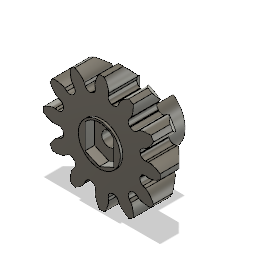
PinionGear (Autodesk Fusion 360 design; units mm, degrees)
description: Spur Gear; Module: 1.75; Num Teeth: 12; Pressure Angle: 20.0; Backlash: 0.00 mm
Autodesk Fusion 360 part; units mm, degrees
(part 1 of 3)
sketch "Sketch1" plane through (0, 0, 0) normal (0, 0, 1) x (1, 0, 0) in component "Spur Gear (12 teeth)"
  circle A0 centre (0, 0) radius 8.3492
  circle A1 centre (0, 0) radius 3
extrude "Extrude1" add sketch "Sketch1" along normal blind 6 in component "Spur Gear (12 teeth)"
sketch "Sketch2" plane through (0, 0, 0) normal (0, 0, 1) x (1, 0, 0) in component "Spur Gear (12 teeth)"
  spline S0 degree 5 poles (9.7621, -1.4335) (9.7691, -1.4345) (9.783, -1.4364) (9.8041, -1.4384) (9.8322, -1.4399) (9.8676, -1.44) (9.903, -1.4389) (9.9385, -1.437) (9.9741, -1.4347) (10.0097, -1.4321) (10.0453, -1.4292) (10.081, -1.4258) (10.1167, -1.422) (10.1525, -1.4175) (10.1882, -1.4124) (10.224, -1.4067) (10.2599, -1.4005) (10.2957, -1.3939) (10.3316, -1.387) (10.3674, -1.3797) (10.4033, -1.3721) (10.4391, -1.364) (10.475, -1.3556) (10.5109, -1.3469) (10.5468, -1.3377) (10.5826, -1.3281) (10.6185, -1.3182) (10.6543, -1.3079) (10.6902, -1.2973) (10.726, -1.2864) (10.7619, -1.2752) (10.7977, -1.2636) (10.8335, -1.2517) (10.8693, -1.2395) (10.905, -1.227) (10.9408, -1.2141) (10.9765, -1.2009) (11.0122, -1.1875) (11.0479, -1.1737) (11.0835, -1.1597) (11.1191, -1.1453) (11.1547, -1.1307) (11.1903, -1.1158) (11.2259, -1.1005) (11.2614, -1.085) (11.2968, -1.0692) (11.3323, -1.0532) (11.3677, -1.0368) (11.4031, -1.0202) (11.4384, -1.0033) (11.4737, -0.9861) (11.5089, -0.9687) (11.5441, -0.951) (11.5793, -0.933) (11.6144, -0.9148) (11.6495, -0.8963) (11.6845, -0.8775) (11.7195, -0.8585) (11.7545, -0.8392) (11.7894, -0.8197) (11.8242, -0.7999) (11.859, -0.7799) (11.8937, -0.7596) (11.9284, -0.7391) (11.963, -0.7183) (11.9976, -0.6972) (12.0321, -0.6759) (12.0666, -0.6544) (12.101, -0.6327) (12.1353, -0.6106) (12.1696, -0.5884) (12.197, -0.5704) (12.2175, -0.5568) (12.2311, -0.5477) (12.238, -0.5431) knots 0 0 0 0 0 0 0.01428571 0.02857143 0.04285714 0.05714286 0.07142857 0.08571429 0.1 0.11428571 0.12857143 0.14285714 0.15714286 0.17142857 0.18571429 0.2 0.21428571 0.22857143 0.24285714 0.25714286 0.27142857 0.28571429 0.3 0.31428571 0.32857143 0.34285714 0.35714286 0.37142857 0.38571429 0.4 0.41428571 0.42857143 0.44285714 0.45714286 0.47142857 0.48571429 0.5 0.51428571 0.52857143 0.54285714 0.55714286 0.57142857 0.58571429 0.6 0.61428571 0.62857143 0.64285714 0.65714286 0.67142857 0.68571429 0.7 0.71428571 0.72857143 0.74285714 0.75714286 0.77142857 0.78571429 0.8 0.81428571 0.82857143 0.84285714 0.85714286 0.87142857 0.88571429 0.9 0.91428571 0.92857143 0.94285714 0.95714286 0.97142857 0.98571429 1 1 1 1 1 1
  spline S1 degree 5 poles (9.7621, 1.4335) (9.7691, 1.4345) (9.783, 1.4364) (9.8041, 1.4384) (9.8322, 1.4399) (9.8676, 1.44) (9.903, 1.4389) (9.9385, 1.437) (9.9741, 1.4347) (10.0097, 1.4321) (10.0453, 1.4292) (10.081, 1.4258) (10.1167, 1.422) (10.1525, 1.4175) (10.1882, 1.4124) (10.224, 1.4067) (10.2599, 1.4005) (10.2957, 1.3939) (10.3316, 1.387) (10.3674, 1.3797) (10.4033, 1.3721) (10.4391, 1.364) (10.475, 1.3556) (10.5109, 1.3469) (10.5468, 1.3377) (10.5826, 1.3281) (10.6185, 1.3182) (10.6543, 1.3079) (10.6902, 1.2973) (10.726, 1.2864) (10.7619, 1.2752) (10.7977, 1.2636) (10.8335, 1.2517) (10.8693, 1.2395) (10.905, 1.227) (10.9408, 1.2141) (10.9765, 1.2009) (11.0122, 1.1875) (11.0479, 1.1737) (11.0835, 1.1597) (11.1191, 1.1453) (11.1547, 1.1307) (11.1903, 1.1158) (11.2259, 1.1005) (11.2614, 1.085) (11.2968, 1.0692) (11.3323, 1.0532) (11.3677, 1.0368) (11.4031, 1.0202) (11.4384, 1.0033) (11.4737, 0.9861) (11.5089, 0.9687) (11.5441, 0.951) (11.5793, 0.933) (11.6144, 0.9148) (11.6495, 0.8963) (11.6845, 0.8775) (11.7195, 0.8585) (11.7545, 0.8392) (11.7894, 0.8197) (11.8242, 0.7999) (11.859, 0.7799) (11.8937, 0.7596) (11.9284, 0.7391) (11.963, 0.7183) (11.9976, 0.6972) (12.0321, 0.6759) (12.0666, 0.6544) (12.101, 0.6327) (12.1353, 0.6106) (12.1696, 0.5884) (12.197, 0.5704) (12.2175, 0.5568) (12.2311, 0.5477) (12.238, 0.5431) knots 0 0 0 0 0 0 0.01428571 0.02857143 0.04285714 0.05714286 0.07142857 0.08571429 0.1 0.11428571 0.12857143 0.14285714 0.15714286 0.17142857 0.18571429 0.2 0.21428571 0.22857143 0.24285714 0.25714286 0.27142857 0.28571429 0.3 0.31428571 0.32857143 0.34285714 0.35714286 0.37142857 0.38571429 0.4 0.41428571 0.42857143 0.44285714 0.45714286 0.47142857 0.48571429 0.5 0.51428571 0.52857143 0.54285714 0.55714286 0.57142857 0.58571429 0.6 0.61428571 0.62857143 0.64285714 0.65714286 0.67142857 0.68571429 0.7 0.71428571 0.72857143 0.74285714 0.75714286 0.77142857 0.78571429 0.8 0.81428571 0.82857143 0.84285714 0.85714286 0.87142857 0.88571429 0.9 0.91428571 0.92857143 0.94285714 0.95714286 0.97142857 0.98571429 1 1 1 1 1 1
  arc A0 (12.238, -0.5431) -> (12.238, 0.5431) centre (0, 0) ccw
  line L0 (8.2507, -1.213) -> (9.7621, -1.4335)
  line L1 (8.2507, 1.213) -> (9.7621, 1.4335)
  line L2 (8.2507, -1.213) -> (8.2507, 1.213)
  point P0 (9.9336, -1.4372)
  point P1 (10.1076, -1.4229)
  point P2 (10.2831, -1.3962)
  point P3 (10.4598, -1.3592)
  point P4 (10.6372, -1.3128)
  point P5 (10.8153, -1.2577)
  point P6 (10.9937, -1.1944)
  point P7 (11.1723, -1.1233)
  point P8 (11.3509, -1.0445)
  point P9 (11.5293, -0.9584)
  point P10 (11.7074, -0.8651)
  point P11 (11.885, -0.7647)
  point P12 (12.0619, -0.6573)
  point P13 (9.9336, 1.4372)
  point P14 (10.1076, 1.4229)
  point P15 (10.2831, 1.3962)
  point P16 (10.4598, 1.3592)
  point P17 (10.6372, 1.3128)
  point P18 (10.8153, 1.2577)
  point P19 (10.9937, 1.1944)
  point P20 (11.1723, 1.1233)
  point P21 (11.3509, 1.0445)
  point P22 (11.5293, 0.9584)
  point P23 (11.7074, 0.8651)
  point P24 (11.885, 0.7647)
  point P25 (12.0619, 0.6573)
extrude "Extrude2" add sketch "Sketch2" along normal blind 6 in component "Spur Gear (12 teeth)"
fillet "Fillet1" radius 1 2 edges at (8.2604, -1.2145, 3) (8.2604, 1.2145, 3) in component "Spur Gear (12 teeth)"
pattern_circular "C-Pattern1" count 12 over 360 about axis through (0, 0, 0) along (0, 0, 1) of "Extrude2", "Fillet1" in component "Spur Gear (12 teeth)"
sketch "Sketch3" plane through (0, 0, 0) normal (0, 0, 1) x (1, 0, 0) in component "Spur Gear (12 teeth)"
  circle A0 centre (0, 0) radius 10.5 construction
  circle A1 centre (0, 0) radius 12.25 construction
  point P0 (0.5431, 12.238)
  constraint concentric A0 A1
  constraint coincident A1 P0
sketch "Sketch1 (2)" plane through (0, 0, 0) normal (0, 1, 0) x (1, 0, 0)
  line L0 (-12.25, 0) -> (12.25, 0) construction
  line L1 (12.25, 0) -> (12.25, -2)
  line L2 (12.25, -2) -> (10.25, 0)
  line L3 (0, 0) -> (0, 10) construction
  line L4 (10.25, 0) -> (12.25, 0)
  dimension "d8" = 2
  constraint coincident L0.end L1.start
  constraint perpendicular L0 L1
  constraint coincident L0 L2.end
  constraint coincident L3.start origin
  constraint perpendicular L0 L3
  constraint equal L1 L4
  measures "d8" distance of L0.end L1.end
revolve "Revolve1" cut sketch "Sketch1 (2)" angle 360 about axis through (0, 0, 0) along (0, 0, -1) in component "Spur Gear (12 teeth)"
sketch "Sketch3 (2)" plane through (0, 0, 0) normal (0, 0, -1) x (-1, 0, 0)
  arc A0 (-9.5002, -3.8482) -> (-8.0827, -6.3033) centre (0, 0) ccw
  spline S0 degree 5 poles (-7.7374, -6.1225) (-7.743, -6.1269) (-7.7542, -6.1354) (-7.7714, -6.1477) (-7.795, -6.1631) (-7.8255, -6.1809) (-7.8568, -6.1976) (-7.8885, -6.2138) (-7.9205, -6.2295) (-7.9526, -6.2451) (-7.9849, -6.2604) (-8.0173, -6.2752) (-8.0434, -6.2868) (-8.0631, -6.2952) (-8.0763, -6.3006) (-8.0827, -6.3033) knots 0 0 0 0 0 0 0.014286 0.028571 0.042857 0.057143 0.071429 0.085714 0.1 0.114286 0.128571 0.142857 0.156761 0.156761 0.156761 0.156761 0.156761 0.156761
  line L0 (-7.7374, -6.1225) -> (-7.2884, -5.7679)
  arc A1 (-5.9553, -5.8518) -> (-7.2884, -5.7679) centre (-6.6686, -6.5526) ccw
  arc A2 (-5.9553, -5.8518) -> (-5.8518, -5.9553) centre (0, 0) ccw
  arc A3 (-5.7679, -7.2884) -> (-5.8518, -5.9553) centre (-6.5526, -6.6686) ccw
  line L1 (-5.7679, -7.2884) -> (-6.1225, -7.7374)
  spline S1 degree 5 poles (-6.1225, -7.7374) (-6.1269, -7.743) (-6.1354, -7.7542) (-6.1477, -7.7714) (-6.1631, -7.795) (-6.1809, -7.8255) (-6.1976, -7.8568) (-6.2138, -7.8885) (-6.2295, -7.9205) (-6.2451, -7.9526) (-6.2604, -7.9849) (-6.2752, -8.0173) (-6.2868, -8.0434) (-6.2952, -8.0631) (-6.3006, -8.0763) (-6.3033, -8.0827) knots 0 0 0 0 0 0 0.014286 0.028571 0.042857 0.057143 0.071429 0.085714 0.1 0.114286 0.128571 0.142857 0.156761 0.156761 0.156761 0.156761 0.156761 0.156761
  arc A4 (-6.3033, -8.0827) -> (-3.8482, -9.5002) centre (0, 0) ccw
  spline S2 degree 5 poles (-3.6396, -9.171) (-3.6422, -9.1775) (-3.6476, -9.1905) (-3.6563, -9.2098) (-3.6691, -9.2349) (-3.6867, -9.2656) (-3.7054, -9.2957) (-3.7248, -9.3255) (-3.7446, -9.3552) (-3.7646, -9.3847) (-3.785, -9.4141) (-3.8056, -9.4432) (-3.8224, -9.4662) (-3.8353, -9.4833) (-3.8439, -9.4946) (-3.8482, -9.5002) knots 0 0 0 0 0 0 0.014286 0.028571 0.042857 0.057143 0.071429 0.085714 0.1 0.114286 0.128571 0.142857 0.156761 0.156761 0.156761 0.156761 0.156761 0.156761
  line L2 (-3.6396, -9.171) -> (-3.428, -8.6393)
  arc A5 (-2.2316, -8.0454) -> (-3.428, -8.6393) centre (-2.4989, -9.0091) ccw
  arc A6 (-2.2316, -8.0454) -> (-2.0901, -8.0834) centre (0, 0) ccw
  arc A7 (-1.3509, -9.1959) -> (-2.0901, -8.0834) centre (-2.3404, -9.0515) ccw
  line L3 (-1.3509, -9.1959) -> (-1.4335, -9.7621)
  spline S3 degree 5 poles (-1.4335, -9.7621) (-1.4345, -9.7691) (-1.4364, -9.783) (-1.4384, -9.8041) (-1.4399, -9.8322) (-1.44, -9.8676) (-1.4389, -9.903) (-1.437, -9.9385) (-1.4347, -9.9741) (-1.4321, -10.0097) (-1.4292, -10.0453) (-1.4258, -10.0808) (-1.4228, -10.1092) (-1.4202, -10.1304) (-1.4184, -10.1446) (-1.4175, -10.1515) knots 0 0 0 0 0 0 0.014286 0.028571 0.042857 0.057143 0.071429 0.085714 0.1 0.114286 0.128571 0.142857 0.156761 0.156761 0.156761 0.156761 0.156761 0.156761
  arc A8 (-1.4175, -10.1515) -> (1.4175, -10.1515) centre (0, 0) ccw
  spline S4 degree 5 poles (1.4335, -9.7621) (1.4345, -9.7691) (1.4364, -9.783) (1.4384, -9.8041) (1.4399, -9.8322) (1.44, -9.8676) (1.4389, -9.903) (1.437, -9.9385) (1.4347, -9.9741) (1.4321, -10.0097) (1.4292, -10.0453) (1.4258, -10.0808) (1.4228, -10.1092) (1.4202, -10.1304) (1.4184, -10.1446) (1.4175, -10.1515) knots 0 0 0 0 0 0 0.014286 0.028571 0.042857 0.057143 0.071429 0.085714 0.1 0.114286 0.128571 0.142857 0.156761 0.156761 0.156761 0.156761 0.156761 0.156761
  line L4 (1.4335, -9.7621) -> (1.3509, -9.1959)
  arc A9 (2.0901, -8.0834) -> (1.3509, -9.1959) centre (2.3404, -9.0515) ccw
  arc A10 (2.0901, -8.0834) -> (2.2316, -8.0454) centre (0, 0) ccw
  arc A11 (3.428, -8.6393) -> (2.2316, -8.0454) centre (2.4989, -9.0091) ccw
  line L5 (3.428, -8.6393) -> (3.6396, -9.171)
  spline S5 degree 5 poles (3.6396, -9.171) (3.6422, -9.1775) (3.6476, -9.1905) (3.6563, -9.2098) (3.6691, -9.2349) (3.6867, -9.2656) (3.7054, -9.2957) (3.7248, -9.3255) (3.7446, -9.3552) (3.7646, -9.3847) (3.785, -9.4141) (3.8056, -9.4432) (3.8224, -9.4662) (3.8353, -9.4833) (3.8439, -9.4946) (3.8482, -9.5002) knots 0 0 0 0 0 0 0.014286 0.028571 0.042857 0.057143 0.071429 0.085714 0.1 0.114286 0.128571 0.142857 0.156761 0.156761 0.156761 0.156761 0.156761 0.156761
  arc A12 (3.8482, -9.5002) -> (6.3033, -8.0827) centre (0, 0) ccw
  spline S6 degree 5 poles (6.1225, -7.7374) (6.1269, -7.743) (6.1354, -7.7542) (6.1477, -7.7714) (6.1631, -7.795) (6.1809, -7.8255) (6.1976, -7.8568) (6.2138, -7.8885) (6.2295, -7.9205) (6.2451, -7.9526) (6.2604, -7.9849) (6.2752, -8.0173) (6.2868, -8.0434) (6.2952, -8.0631) (6.3006, -8.0763) (6.3033, -8.0827) knots 0 0 0 0 0 0 0.014286 0.028571 0.042857 0.057143 0.071429 0.085714 0.1 0.114286 0.128571 0.142857 0.156761 0.156761 0.156761 0.156761 0.156761 0.156761
  line L6 (6.1225, -7.7374) -> (5.7679, -7.2884)
  arc A13 (5.8518, -5.9553) -> (5.7679, -7.2884) centre (6.5526, -6.6686) ccw
  arc A14 (5.8518, -5.9553) -> (5.9553, -5.8518) centre (0, 0) ccw
  arc A15 (7.2884, -5.7679) -> (5.9553, -5.8518) centre (6.6686, -6.5526) ccw
  line L7 (7.2884, -5.7679) -> (7.7374, -6.1225)
  spline S7 degree 5 poles (7.7374, -6.1225) (7.743, -6.1269) (7.7542, -6.1354) (7.7714, -6.1477) (7.795, -6.1631) (7.8255, -6.1809) (7.8568, -6.1976) (7.8885, -6.2138) (7.9205, -6.2295) (7.9526, -6.2451) (7.9849, -6.2604) (8.0173, -6.2752) (8.0434, -6.2868) (8.0631, -6.2952) (8.0763, -6.3006) (8.0827, -6.3033) knots 0 0 0 0 0 0 0.014286 0.028571 0.042857 0.057143 0.071429 0.085714 0.1 0.114286 0.128571 0.142857 0.156761 0.156761 0.156761 0.156761 0.156761 0.156761
  arc A16 (8.0827, -6.3033) -> (9.5002, -3.8482) centre (0, 0) ccw
  spline S8 degree 5 poles (9.171, -3.6396) (9.1775, -3.6422) (9.1905, -3.6476) (9.2098, -3.6563) (9.2349, -3.6691) (9.2656, -3.6867) (9.2957, -3.7054) (9.3255, -3.7248) (9.3552, -3.7446) (9.3847, -3.7646) (9.4141, -3.785) (9.4432, -3.8056) (9.4662, -3.8224) (9.4833, -3.8353) (9.4946, -3.8439) (9.5002, -3.8482) knots 0 0 0 0 0 0 0.014286 0.028571 0.042857 0.057143 0.071429 0.085714 0.1 0.114286 0.128571 0.142857 0.156761 0.156761 0.156761 0.156761 0.156761 0.156761
  line L8 (9.171, -3.6396) -> (8.6393, -3.428)
  arc A17 (8.0454, -2.2316) -> (8.6393, -3.428) centre (9.0091, -2.4989) ccw
  arc A18 (8.0454, -2.2316) -> (8.0834, -2.0901) centre (0, 0) ccw
  arc A19 (9.1959, -1.3509) -> (8.0834, -2.0901) centre (9.0515, -2.3404) ccw
  line L9 (9.1959, -1.3509) -> (9.7621, -1.4335)
  spline S9 degree 5 poles (9.7621, -1.4335) (9.7691, -1.4345) (9.783, -1.4364) (9.8041, -1.4384) (9.8322, -1.4399) (9.8676, -1.44) (9.903, -1.4389) (9.9385, -1.437) (9.9741, -1.4347) (10.0097, -1.4321) (10.0453, -1.4292) (10.0808, -1.4258) (10.1092, -1.4228) (10.1304, -1.4202) (10.1446, -1.4184) (10.1515, -1.4175) knots 0 0 0 0 0 0 0.014286 0.028571 0.042857 0.057143 0.071429 0.085714 0.1 0.114286 0.128571 0.142857 0.156761 0.156761 0.156761 0.156761 0.156761 0.156761
  arc A20 (10.1515, -1.4175) -> (10.1515, 1.4175) centre (0, 0) ccw
  spline S10 degree 5 poles (9.7621, 1.4335) (9.7691, 1.4345) (9.783, 1.4364) (9.8041, 1.4384) (9.8322, 1.4399) (9.8676, 1.44) (9.903, 1.4389) (9.9385, 1.437) (9.9741, 1.4347) (10.0097, 1.4321) (10.0453, 1.4292) (10.0808, 1.4258) (10.1092, 1.4228) (10.1304, 1.4202) (10.1446, 1.4184) (10.1515, 1.4175) knots 0 0 0 0 0 0 0.014286 0.028571 0.042857 0.057143 0.071429 0.085714 0.1 0.114286 0.128571 0.142857 0.156761 0.156761 0.156761 0.156761 0.156761 0.156761
  line L10 (9.7621, 1.4335) -> (9.1959, 1.3509)
  arc A21 (8.0834, 2.0901) -> (9.1959, 1.3509) centre (9.0515, 2.3404) ccw
  arc A22 (8.0834, 2.0901) -> (8.0454, 2.2316) centre (0, 0) ccw
  arc A23 (8.6393, 3.428) -> (8.0454, 2.2316) centre (9.0091, 2.4989) ccw
  line L11 (8.6393, 3.428) -> (9.171, 3.6396)
  spline S11 degree 5 poles (9.171, 3.6396) (9.1775, 3.6422) (9.1905, 3.6476) (9.2098, 3.6563) (9.2349, 3.6691) (9.2656, 3.6867) (9.2957, 3.7054) (9.3255, 3.7248) (9.3552, 3.7446) (9.3847, 3.7646) (9.4141, 3.785) (9.4432, 3.8056) (9.4662, 3.8224) (9.4833, 3.8353) (9.4946, 3.8439) (9.5002, 3.8482) knots 0 0 0 0 0 0 0.014286 0.028571 0.042857 0.057143 0.071429 0.085714 0.1 0.114286 0.128571 0.142857 0.156761 0.156761 0.156761 0.156761 0.156761 0.156761
  arc A24 (9.5002, 3.8482) -> (8.0827, 6.3033) centre (0, 0) ccw
  spline S12 degree 5 poles (7.7374, 6.1225) (7.743, 6.1269) (7.7542, 6.1354) (7.7714, 6.1477) (7.795, 6.1631) (7.8255, 6.1809) (7.8568, 6.1976) (7.8885, 6.2138) (7.9205, 6.2295) (7.9526, 6.2451) (7.9849, 6.2604) (8.0173, 6.2752) (8.0434, 6.2868) (8.0631, 6.2952) (8.0763, 6.3006) (8.0827, 6.3033) knots 0 0 0 0 0 0 0.014286 0.028571 0.042857 0.057143 0.071429 0.085714 0.1 0.114286 0.128571 0.142857 0.156761 0.156761 0.156761 0.156761 0.156761 0.156761
  line L12 (7.7374, 6.1225) -> (7.2884, 5.7679)
  arc A25 (5.9553, 5.8518) -> (7.2884, 5.7679) centre (6.6686, 6.5526) ccw
  arc A26 (5.9553, 5.8518) -> (5.8518, 5.9553) centre (0, 0) ccw
  arc A27 (5.7679, 7.2884) -> (5.8518, 5.9553) centre (6.5526, 6.6686) ccw
  line L13 (5.7679, 7.2884) -> (6.1225, 7.7374)
  spline S13 degree 5 poles (6.1225, 7.7374) (6.1269, 7.743) (6.1354, 7.7542) (6.1477, 7.7714) (6.1631, 7.795) (6.1809, 7.8255) (6.1976, 7.8568) (6.2138, 7.8885) (6.2295, 7.9205) (6.2451, 7.9526) (6.2604, 7.9849) (6.2752, 8.0173) (6.2868, 8.0434) (6.2952, 8.0631) (6.3006, 8.0763) (6.3033, 8.0827) knots 0 0 0 0 0 0 0.014286 0.028571 0.042857 0.057143 0.071429 0.085714 0.1 0.114286 0.128571 0.142857 0.156761 0.156761 0.156761 0.156761 0.156761 0.156761
  arc A28 (6.3033, 8.0827) -> (3.8482, 9.5002) centre (0, 0) ccw
  spline S14 degree 5 poles (3.6396, 9.171) (3.6422, 9.1775) (3.6476, 9.1905) (3.6563, 9.2098) (3.6691, 9.2349) (3.6867, 9.2656) (3.7054, 9.2957) (3.7248, 9.3255) (3.7446, 9.3552) (3.7646, 9.3847) (3.785, 9.4141) (3.8056, 9.4432) (3.8224, 9.4662) (3.8353, 9.4833) (3.8439, 9.4946) (3.8482, 9.5002) knots 0 0 0 0 0 0 0.014286 0.028571 0.042857 0.057143 0.071429 0.085714 0.1 0.114286 0.128571 0.142857 0.156761 0.156761 0.156761 0.156761 0.156761 0.156761
  line L14 (3.6396, 9.171) -> (3.428, 8.6393)
  arc A29 (2.2316, 8.0454) -> (3.428, 8.6393) centre (2.4989, 9.0091) ccw
  arc A30 (2.2316, 8.0454) -> (2.0901, 8.0834) centre (0, 0) ccw
  arc A31 (1.3509, 9.1959) -> (2.0901, 8.0834) centre (2.3404, 9.0515) ccw
  line L15 (1.3509, 9.1959) -> (1.4335, 9.7621)
  spline S15 degree 5 poles (1.4335, 9.7621) (1.4345, 9.7691) (1.4364, 9.783) (1.4384, 9.8041) (1.4399, 9.8322) (1.44, 9.8676) (1.4389, 9.903) (1.437, 9.9385) (1.4347, 9.9741) (1.4321, 10.0097) (1.4292, 10.0453) (1.4258, 10.0808) (1.4228, 10.1092) (1.4202, 10.1304) (1.4184, 10.1446) (1.4175, 10.1515) knots 0 0 0 0 0 0 0.014286 0.028571 0.042857 0.057143 0.071429 0.085714 0.1 0.114286 0.128571 0.142857 0.156761 0.156761 0.156761 0.156761 0.156761 0.156761
  arc A32 (1.4175, 10.1515) -> (-1.4175, 10.1515) centre (0, 0) ccw
  spline S16 degree 5 poles (-1.4335, 9.7621) (-1.4345, 9.7691) (-1.4364, 9.783) (-1.4384, 9.8041) (-1.4399, 9.8322) (-1.44, 9.8676) (-1.4389, 9.903) (-1.437, 9.9385) (-1.4347, 9.9741) (-1.4321, 10.0097) (-1.4292, 10.0453) (-1.4258, 10.0808) (-1.4228, 10.1092) (-1.4202, 10.1304) (-1.4184, 10.1446) (-1.4175, 10.1515) knots 0 0 0 0 0 0 0.014286 0.028571 0.042857 0.057143 0.071429 0.085714 0.1 0.114286 0.128571 0.142857 0.156761 0.156761 0.156761 0.156761 0.156761 0.156761
  line L16 (-1.4335, 9.7621) -> (-1.3509, 9.1959)
  arc A33 (-2.0901, 8.0834) -> (-1.3509, 9.1959) centre (-2.3404, 9.0515) ccw
  arc A34 (-2.0901, 8.0834) -> (-2.2316, 8.0454) centre (0, 0) ccw
  arc A35 (-3.428, 8.6393) -> (-2.2316, 8.0454) centre (-2.4989, 9.0091) ccw
  line L17 (-3.428, 8.6393) -> (-3.6396, 9.171)
  spline S17 degree 5 poles (-3.6396, 9.171) (-3.6422, 9.1775) (-3.6476, 9.1905) (-3.6563, 9.2098) (-3.6691, 9.2349) (-3.6867, 9.2656) (-3.7054, 9.2957) (-3.7248, 9.3255) (-3.7446, 9.3552) (-3.7646, 9.3847) (-3.785, 9.4141) (-3.8056, 9.4432) (-3.8224, 9.4662) (-3.8353, 9.4833) (-3.8439, 9.4946) (-3.8482, 9.5002) knots 0 0 0 0 0 0 0.014286 0.028571 0.042857 0.057143 0.071429 0.085714 0.1 0.114286 0.128571 0.142857 0.156761 0.156761 0.156761 0.156761 0.156761 0.156761
  arc A36 (-3.8482, 9.5002) -> (-6.3033, 8.0827) centre (0, 0) ccw
  spline S18 degree 5 poles (-6.1225, 7.7374) (-6.1269, 7.743) (-6.1354, 7.7542) (-6.1477, 7.7714) (-6.1631, 7.795) (-6.1809, 7.8255) (-6.1976, 7.8568) (-6.2138, 7.8885) (-6.2295, 7.9205) (-6.2451, 7.9526) (-6.2604, 7.9849) (-6.2752, 8.0173) (-6.2868, 8.0434) (-6.2952, 8.0631) (-6.3006, 8.0763) (-6.3033, 8.0827) knots 0 0 0 0 0 0 0.014286 0.028571 0.042857 0.057143 0.071429 0.085714 0.1 0.114286 0.128571 0.142857 0.156761 0.156761 0.156761 0.156761 0.156761 0.156761
  line L18 (-6.1225, 7.7374) -> (-5.7679, 7.2884)
  arc A37 (-5.8518, 5.9553) -> (-5.7679, 7.2884) centre (-6.5526, 6.6686) ccw
  arc A38 (-5.8518, 5.9553) -> (-5.9553, 5.8518) centre (0, 0) ccw
  arc A39 (-7.2884, 5.7679) -> (-5.9553, 5.8518) centre (-6.6686, 6.5526) ccw
  line L19 (-7.2884, 5.7679) -> (-7.7374, 6.1225)
  spline S19 degree 5 poles (-7.7374, 6.1225) (-7.743, 6.1269) (-7.7542, 6.1354) (-7.7714, 6.1477) (-7.795, 6.1631) (-7.8255, 6.1809) (-7.8568, 6.1976) (-7.8885, 6.2138) (-7.9205, 6.2295) (-7.9526, 6.2451) (-7.9849, 6.2604) (-8.0173, 6.2752) (-8.0434, 6.2868) (-8.0631, 6.2952) (-8.0763, 6.3006) (-8.0827, 6.3033) knots 0 0 0 0 0 0 0.014286 0.028571 0.042857 0.057143 0.071429 0.085714 0.1 0.114286 0.128571 0.142857 0.156761 0.156761 0.156761 0.156761 0.156761 0.156761
  arc A40 (-8.0827, 6.3033) -> (-9.5002, 3.8482) centre (0, 0) ccw
  spline S20 degree 5 poles (-9.171, 3.6396) (-9.1775, 3.6422) (-9.1905, 3.6476) (-9.2098, 3.6563) (-9.2349, 3.6691) (-9.2656, 3.6867) (-9.2957, 3.7054) (-9.3255, 3.7248) (-9.3552, 3.7446) (-9.3847, 3.7646) (-9.4141, 3.785) (-9.4432, 3.8056) (-9.4662, 3.8224) (-9.4833, 3.8353) (-9.4946, 3.8439) (-9.5002, 3.8482) knots 0 0 0 0 0 0 0.014286 0.028571 0.042857 0.057143 0.071429 0.085714 0.1 0.114286 0.128571 0.142857 0.156761 0.156761 0.156761 0.156761 0.156761 0.156761
  line L20 (-9.171, 3.6396) -> (-8.6393, 3.428)
  arc A41 (-8.0454, 2.2316) -> (-8.6393, 3.428) centre (-9.0091, 2.4989) ccw
  arc A42 (-8.0454, 2.2316) -> (-8.0834, 2.0901) centre (0, 0) ccw
  arc A43 (-9.1959, 1.3509) -> (-8.0834, 2.0901) centre (-9.0515, 2.3404) ccw
  line L21 (-9.1959, 1.3509) -> (-9.7621, 1.4335)
  spline S21 degree 5 poles (-9.7621, 1.4335) (-9.7691, 1.4345) (-9.783, 1.4364) (-9.8041, 1.4384) (-9.8322, 1.4399) (-9.8676, 1.44) (-9.903, 1.4389) (-9.9385, 1.437) (-9.9741, 1.4347) (-10.0097, 1.4321) (-10.0453, 1.4292) (-10.0808, 1.4258) (-10.1092, 1.4228) (-10.1304, 1.4202) (-10.1446, 1.4184) (-10.1515, 1.4175) knots 0 0 0 0 0 0 0.014286 0.028571 0.042857 0.057143 0.071429 0.085714 0.1 0.114286 0.128571 0.142857 0.156761 0.156761 0.156761 0.156761 0.156761 0.156761
  arc A44 (-10.1515, 1.4175) -> (-10.1515, -1.4175) centre (0, 0) ccw
  spline S22 degree 5 poles (-9.7621, -1.4335) (-9.7691, -1.4345) (-9.783, -1.4364) (-9.8041, -1.4384) (-9.8322, -1.4399) (-9.8676, -1.44) (-9.903, -1.4389) (-9.9385, -1.437) (-9.9741, -1.4347) (-10.0097, -1.4321) (-10.0453, -1.4292) (-10.0808, -1.4258) (-10.1092, -1.4228) (-10.1304, -1.4202) (-10.1446, -1.4184) (-10.1515, -1.4175) knots 0 0 0 0 0 0 0.014286 0.028571 0.042857 0.057143 0.071429 0.085714 0.1 0.114286 0.128571 0.142857 0.156761 0.156761 0.156761 0.156761 0.156761 0.156761
  line L22 (-9.7621, -1.4335) -> (-9.1959, -1.3509)
  arc A45 (-8.0834, -2.0901) -> (-9.1959, -1.3509) centre (-9.0515, -2.3404) ccw
  arc A46 (-8.0834, -2.0901) -> (-8.0454, -2.2316) centre (0, 0) ccw
  arc A47 (-8.6393, -3.428) -> (-8.0454, -2.2316) centre (-9.0091, -2.4989) ccw
  line L23 (-8.6393, -3.428) -> (-9.171, -3.6396)
  spline S23 degree 5 poles (-9.171, -3.6396) (-9.1775, -3.6422) (-9.1905, -3.6476) (-9.2098, -3.6563) (-9.2349, -3.6691) (-9.2656, -3.6867) (-9.2957, -3.7054) (-9.3255, -3.7248) (-9.3552, -3.7446) (-9.3847, -3.7646) (-9.4141, -3.785) (-9.4432, -3.8056) (-9.4662, -3.8224) (-9.4833, -3.8353) (-9.4946, -3.8439) (-9.5002, -3.8482) knots 0 0 0 0 0 0 0.014286 0.028571 0.042857 0.057143 0.071429 0.085714 0.1 0.114286 0.128571 0.142857 0.156761 0.156761 0.156761 0.156761 0.156761 0.156761
  circle A48 centre (0, 0) radius 3
  circle A49 centre (0, 0) radius 6
  dimension "d10" = 12
  constraint concentric A0 A49
  measures "d10" diameter of A49
extrude "Extrude3" add sketch "Sketch3 (2)" along normal blind 5.5 contours A48 | A49 in component "Spur Gear (12 teeth)"
sketch "Sketch4" plane through (0, 0, -5.5) normal (0, 0, -1) x (-1, 0, 0)
  circle A0 centre (0, 0) radius 6
  line L0 (-3.5, 4.6) -> (3.5, 4.6) construction
  line L1 (3.5, 4.6) -> (3.5, -4.6) construction
  line L2 (3.5, -4.6) -> (-3.5, -4.6) construction
  line L3 (-3.5, -4.6) -> (-3.5, 4.6) construction
  line L4 (-3.5, 4.6) -> (3.5, -4.6) construction
  line L5 (3.5, 4.6) -> (-3.5, -4.6) construction
  line L6 (-3.5, -4.6) -> (-3.5, 4.8734)
  line L7 (3.5, -4.6) -> (3.5, 4.8734)
  line L8 (-3.5, -4.6) -> (3.5, -4.6)
  line L9 (-3.5, -2.6) -> (-1.5, -4.6)
  line L10 (0, 0) -> (0, -7) construction
  line L11 (3.5, -2.6) -> (1.5, -4.6)
  dimension "d13" = 7
  dimension "d14" = 4.6
  dimension "d15" = 45
  dimension "d16" = 2
  constraint perpendicular L0 L1
  constraint parallel L0 L2
  constraint parallel L1 L3
  constraint horizontal L0
  constraint coincident L4 A0.centre
  constraint coincident L5 A0.centre
  constraint coincident A0.centre L10.start
  constraint coincident A0 L6.end
  constraint collinear L3 L6
  constraint coincident A0 L7.end
  constraint collinear L1 L7
  constraint coincident L3 L9.start
  constraint coincident L2 L9.end
  constraint vertical L10
  constraint symmetric L9.start L10 L11.start
  constraint symmetric L9.end L10 L11.end
  measures "d13" distance of L1 L3
  measures "d14" distance of L2 A0.centre
  measures "d15" angle of L8 L9
  measures "d16" distance of L2.end L9.start
extrude "Extrude4" cut sketch "Sketch4" against normal blind 3.5 contours A0 L6 L7 L8 L9 L11 in component "Spur Gear (12 teeth)"
sketch "Sketch5" plane through (0, 0, 0) normal (0, 0, -1) x (-1, 0, 0)
  circle A0 centre (0, 0) radius 6
  arc A1 (-9.5002, -3.8482) -> (-8.0827, -6.3033) centre (0, 0) ccw
  spline S0 degree 5 poles (-7.7374, -6.1225) (-7.743, -6.1269) (-7.7542, -6.1354) (-7.7714, -6.1477) (-7.795, -6.1631) (-7.8255, -6.1809) (-7.8568, -6.1976) (-7.8885, -6.2138) (-7.9205, -6.2295) (-7.9526, -6.2451) (-7.9849, -6.2604) (-8.0173, -6.2752) (-8.0434, -6.2868) (-8.0631, -6.2952) (-8.0763, -6.3006) (-8.0827, -6.3033) knots 0 0 0 0 0 0 0.014286 0.028571 0.042857 0.057143 0.071429 0.085714 0.1 0.114286 0.128571 0.142857 0.156761 0.156761 0.156761 0.156761 0.156761 0.156761
  line L0 (-7.7374, -6.1225) -> (-7.2884, -5.7679)
  arc A2 (-5.9553, -5.8518) -> (-7.2884, -5.7679) centre (-6.6686, -6.5526) ccw
  arc A3 (-5.9553, -5.8518) -> (-5.8518, -5.9553) centre (0, 0) ccw
  arc A4 (-5.7679, -7.2884) -> (-5.8518, -5.9553) centre (-6.5526, -6.6686) ccw
  line L1 (-5.7679, -7.2884) -> (-6.1225, -7.7374)
  spline S1 degree 5 poles (-6.1225, -7.7374) (-6.1269, -7.743) (-6.1354, -7.7542) (-6.1477, -7.7714) (-6.1631, -7.795) (-6.1809, -7.8255) (-6.1976, -7.8568) (-6.2138, -7.8885) (-6.2295, -7.9205) (-6.2451, -7.9526) (-6.2604, -7.9849) (-6.2752, -8.0173) (-6.2868, -8.0434) (-6.2952, -8.0631) (-6.3006, -8.0763) (-6.3033, -8.0827) knots 0 0 0 0 0 0 0.014286 0.028571 0.042857 0.057143 0.071429 0.085714 0.1 0.114286 0.128571 0.142857 0.156761 0.156761 0.156761 0.156761 0.156761 0.156761
  arc A5 (-6.3033, -8.0827) -> (-3.8482, -9.5002) centre (0, 0) ccw
  spline S2 degree 5 poles (-3.6396, -9.171) (-3.6422, -9.1775) (-3.6476, -9.1905) (-3.6563, -9.2098) (-3.6691, -9.2349) (-3.6867, -9.2656) (-3.7054, -9.2957) (-3.7248, -9.3255) (-3.7446, -9.3552) (-3.7646, -9.3847) (-3.785, -9.4141) (-3.8056, -9.4432) (-3.8224, -9.4662) (-3.8353, -9.4833) (-3.8439, -9.4946) (-3.8482, -9.5002) knots 0 0 0 0 0 0 0.014286 0.028571 0.042857 0.057143 0.071429 0.085714 0.1 0.114286 0.128571 0.142857 0.156761 0.156761 0.156761 0.156761 0.156761 0.156761
  line L2 (-3.6396, -9.171) -> (-3.428, -8.6393)
  arc A6 (-2.2316, -8.0454) -> (-3.428, -8.6393) centre (-2.4989, -9.0091) ccw
  arc A7 (-2.2316, -8.0454) -> (-2.0901, -8.0834) centre (0, 0) ccw
  arc A8 (-1.3509, -9.1959) -> (-2.0901, -8.0834) centre (-2.3404, -9.0515) ccw
  line L3 (-1.3509, -9.1959) -> (-1.4335, -9.7621)
  spline S3 degree 5 poles (-1.4335, -9.7621) (-1.4345, -9.7691) (-1.4364, -9.783) (-1.4384, -9.8041) (-1.4399, -9.8322) (-1.44, -9.8676) (-1.4389, -9.903) (-1.437, -9.9385) (-1.4347, -9.9741) (-1.4321, -10.0097) (-1.4292, -10.0453) (-1.4258, -10.0808) (-1.4228, -10.1092) (-1.4202, -10.1304) (-1.4184, -10.1446) (-1.4175, -10.1515) knots 0 0 0 0 0 0 0.014286 0.028571 0.042857 0.057143 0.071429 0.085714 0.1 0.114286 0.128571 0.142857 0.156761 0.156761 0.156761 0.156761 0.156761 0.156761
  arc A9 (-1.4175, -10.1515) -> (1.4175, -10.1515) centre (0, 0) ccw
  spline S4 degree 5 poles (1.4335, -9.7621) (1.4345, -9.7691) (1.4364, -9.783) (1.4384, -9.8041) (1.4399, -9.8322) (1.44, -9.8676) (1.4389, -9.903) (1.437, -9.9385) (1.4347, -9.9741) (1.4321, -10.0097) (1.4292, -10.0453) (1.4258, -10.0808) (1.4228, -10.1092) (1.4202, -10.1304) (1.4184, -10.1446) (1.4175, -10.1515) knots 0 0 0 0 0 0 0.014286 0.028571 0.042857 0.057143 0.071429 0.085714 0.1 0.114286 0.128571 0.142857 0.156761 0.156761 0.156761 0.156761 0.156761 0.156761
  line L4 (1.4335, -9.7621) -> (1.3509, -9.1959)
  arc A10 (2.0901, -8.0834) -> (1.3509, -9.1959) centre (2.3404, -9.0515) ccw
  arc A11 (2.0901, -8.0834) -> (2.2316, -8.0454) centre (0, 0) ccw
  arc A12 (3.428, -8.6393) -> (2.2316, -8.0454) centre (2.4989, -9.0091) ccw
  line L5 (3.428, -8.6393) -> (3.6396, -9.171)
  spline S5 degree 5 poles (3.6396, -9.171) (3.6422, -9.1775) (3.6476, -9.1905) (3.6563, -9.2098) (3.6691, -9.2349) (3.6867, -9.2656) (3.7054, -9.2957) (3.7248, -9.3255) (3.7446, -9.3552) (3.7646, -9.3847) (3.785, -9.4141) (3.8056, -9.4432) (3.8224, -9.4662) (3.8353, -9.4833) (3.8439, -9.4946) (3.8482, -9.5002) knots 0 0 0 0 0 0 0.014286 0.028571 0.042857 0.057143 0.071429 0.085714 0.1 0.114286 0.128571 0.142857 0.156761 0.156761 0.156761 0.156761 0.156761 0.156761
  arc A13 (3.8482, -9.5002) -> (6.3033, -8.0827) centre (0, 0) ccw
  spline S6 degree 5 poles (6.1225, -7.7374) (6.1269, -7.743) (6.1354, -7.7542) (6.1477, -7.7714) (6.1631, -7.795) (6.1809, -7.8255) (6.1976, -7.8568) (6.2138, -7.8885) (6.2295, -7.9205) (6.2451, -7.9526) (6.2604, -7.9849) (6.2752, -8.0173) (6.2868, -8.0434) (6.2952, -8.0631) (6.3006, -8.0763) (6.3033, -8.0827) knots 0 0 0 0 0 0 0.014286 0.028571 0.042857 0.057143 0.071429 0.085714 0.1 0.114286 0.128571 0.142857 0.156761 0.156761 0.156761 0.156761 0.156761 0.156761
  line L6 (6.1225, -7.7374) -> (5.7679, -7.2884)
  arc A14 (5.8518, -5.9553) -> (5.7679, -7.2884) centre (6.5526, -6.6686) ccw
  arc A15 (5.8518, -5.9553) -> (5.9553, -5.8518) centre (0, 0) ccw
  arc A16 (7.2884, -5.7679) -> (5.9553, -5.8518) centre (6.6686, -6.5526) ccw
  line L7 (7.2884, -5.7679) -> (7.7374, -6.1225)
  spline S7 degree 5 poles (7.7374, -6.1225) (7.743, -6.1269) (7.7542, -6.1354) (7.7714, -6.1477) (7.795, -6.1631) (7.8255, -6.1809) (7.8568, -6.1976) (7.8885, -6.2138) (7.9205, -6.2295) (7.9526, -6.2451) (7.9849, -6.2604) (8.0173, -6.2752) (8.0434, -6.2868) (8.0631, -6.2952) (8.0763, -6.3006) (8.0827, -6.3033) knots 0 0 0 0 0 0 0.014286 0.028571 0.042857 0.057143 0.071429 0.085714 0.1 0.114286 0.128571 0.142857 0.156761 0.156761 0.156761 0.156761 0.156761 0.156761
  arc A17 (8.0827, -6.3033) -> (9.5002, -3.8482) centre (0, 0) ccw
  spline S8 degree 5 poles (9.171, -3.6396) (9.1775, -3.6422) (9.1905, -3.6476) (9.2098, -3.6563) (9.2349, -3.6691) (9.2656, -3.6867) (9.2957, -3.7054) (9.3255, -3.7248) (9.3552, -3.7446) (9.3847, -3.7646) (9.4141, -3.785) (9.4432, -3.8056) (9.4662, -3.8224) (9.4833, -3.8353) (9.4946, -3.8439) (9.5002, -3.8482) knots 0 0 0 0 0 0 0.014286 0.028571 0.042857 0.057143 0.071429 0.085714 0.1 0.114286 0.128571 0.142857 0.156761 0.156761 0.156761 0.156761 0.156761 0.156761
  line L8 (9.171, -3.6396) -> (8.6393, -3.428)
  arc A18 (8.0454, -2.2316) -> (8.6393, -3.428) centre (9.0091, -2.4989) ccw
  arc A19 (8.0454, -2.2316) -> (8.0834, -2.0901) centre (0, 0) ccw
  arc A20 (9.1959, -1.3509) -> (8.0834, -2.0901) centre (9.0515, -2.3404) ccw
  line L9 (9.1959, -1.3509) -> (9.7621, -1.4335)
  spline S9 degree 5 poles (9.7621, -1.4335) (9.7691, -1.4345) (9.783, -1.4364) (9.8041, -1.4384) (9.8322, -1.4399) (9.8676, -1.44) (9.903, -1.4389) (9.9385, -1.437) (9.9741, -1.4347) (10.0097, -1.4321) (10.0453, -1.4292) (10.0808, -1.4258) (10.1092, -1.4228) (10.1304, -1.4202) (10.1446, -1.4184) (10.1515, -1.4175) knots 0 0 0 0 0 0 0.014286 0.028571 0.042857 0.057143 0.071429 0.085714 0.1 0.114286 0.128571 0.142857 0.156761 0.156761 0.156761 0.156761 0.156761 0.156761
  arc A21 (10.1515, -1.4175) -> (10.1515, 1.4175) centre (0, 0) ccw
  spline S10 degree 5 poles (9.7621, 1.4335) (9.7691, 1.4345) (9.783, 1.4364) (9.8041, 1.4384) (9.8322, 1.4399) (9.8676, 1.44) (9.903, 1.4389) (9.9385, 1.437) (9.9741, 1.4347) (10.0097, 1.4321) (10.0453, 1.4292) (10.0808, 1.4258) (10.1092, 1.4228) (10.1304, 1.4202) (10.1446, 1.4184) (10.1515, 1.4175) knots 0 0 0 0 0 0 0.014286 0.028571 0.042857 0.057143 0.071429 0.085714 0.1 0.114286 0.128571 0.142857 0.156761 0.156761 0.156761 0.156761 0.156761 0.156761
  line L10 (9.7621, 1.4335) -> (9.1959, 1.3509)
  arc A22 (8.0834, 2.0901) -> (9.1959, 1.3509) centre (9.0515, 2.3404) ccw
  arc A23 (8.0834, 2.0901) -> (8.0454, 2.2316) centre (0, 0) ccw
  arc A24 (8.6393, 3.428) -> (8.0454, 2.2316) centre (9.0091, 2.4989) ccw
  line L11 (8.6393, 3.428) -> (9.171, 3.6396)
  spline S11 degree 5 poles (9.171, 3.6396) (9.1775, 3.6422) (9.1905, 3.6476) (9.2098, 3.6563) (9.2349, 3.6691) (9.2656, 3.6867) (9.2957, 3.7054) (9.3255, 3.7248) (9.3552, 3.7446) (9.3847, 3.7646) (9.4141, 3.785) (9.4432, 3.8056) (9.4662, 3.8224) (9.4833, 3.8353) (9.4946, 3.8439) (9.5002, 3.8482) knots 0 0 0 0 0 0 0.014286 0.028571 0.042857 0.057143 0.071429 0.085714 0.1 0.114286 0.128571 0.142857 0.156761 0.156761 0.156761 0.156761 0.156761 0.156761
  arc A25 (9.5002, 3.8482) -> (8.0827, 6.3033) centre (0, 0) ccw
  spline S12 degree 5 poles (7.7374, 6.1225) (7.743, 6.1269) (7.7542, 6.1354) (7.7714, 6.1477) (7.795, 6.1631) (7.8255, 6.1809) (7.8568, 6.1976) (7.8885, 6.2138) (7.9205, 6.2295) (7.9526, 6.2451) (7.9849, 6.2604) (8.0173, 6.2752) (8.0434, 6.2868) (8.0631, 6.2952) (8.0763, 6.3006) (8.0827, 6.3033) knots 0 0 0 0 0 0 0.014286 0.028571 0.042857 0.057143 0.071429 0.085714 0.1 0.114286 0.128571 0.142857 0.156761 0.156761 0.156761 0.156761 0.156761 0.156761
  line L12 (7.7374, 6.1225) -> (7.2884, 5.7679)
  arc A26 (5.9553, 5.8518) -> (7.2884, 5.7679) centre (6.6686, 6.5526) ccw
  arc A27 (5.9553, 5.8518) -> (5.8518, 5.9553) centre (0, 0) ccw
  arc A28 (5.7679, 7.2884) -> (5.8518, 5.9553) centre (6.5526, 6.6686) ccw
  line L13 (5.7679, 7.2884) -> (6.1225, 7.7374)
  spline S13 degree 5 poles (6.1225, 7.7374) (6.1269, 7.743) (6.1354, 7.7542) (6.1477, 7.7714) (6.1631, 7.795) (6.1809, 7.8255) (6.1976, 7.8568) (6.2138, 7.8885) (6.2295, 7.9205) (6.2451, 7.9526) (6.2604, 7.9849) (6.2752, 8.0173) (6.2868, 8.0434) (6.2952, 8.0631) (6.3006, 8.0763) (6.3033, 8.0827) knots 0 0 0 0 0 0 0.014286 0.028571 0.042857 0.057143 0.071429 0.085714 0.1 0.114286 0.128571 0.142857 0.156761 0.156761 0.156761 0.156761 0.156761 0.156761
  arc A29 (6.3033, 8.0827) -> (3.8482, 9.5002) centre (0, 0) ccw
  spline S14 degree 5 poles (3.6396, 9.171) (3.6422, 9.1775) (3.6476, 9.1905) (3.6563, 9.2098) (3.6691, 9.2349) (3.6867, 9.2656) (3.7054, 9.2957) (3.7248, 9.3255) (3.7446, 9.3552) (3.7646, 9.3847) (3.785, 9.4141) (3.8056, 9.4432) (3.8224, 9.4662) (3.8353, 9.4833) (3.8439, 9.4946) (3.8482, 9.5002) knots 0 0 0 0 0 0 0.014286 0.028571 0.042857 0.057143 0.071429 0.085714 0.1 0.114286 0.128571 0.142857 0.156761 0.156761 0.156761 0.156761 0.156761 0.156761
  line L14 (3.6396, 9.171) -> (3.428, 8.6393)
  arc A30 (2.2316, 8.0454) -> (3.428, 8.6393) centre (2.4989, 9.0091) ccw
  arc A31 (2.2316, 8.0454) -> (2.0901, 8.0834) centre (0, 0) ccw
  arc A32 (1.3509, 9.1959) -> (2.0901, 8.0834) centre (2.3404, 9.0515) ccw
  line L15 (1.3509, 9.1959) -> (1.4335, 9.7621)
  spline S15 degree 5 poles (1.4335, 9.7621) (1.4345, 9.7691) (1.4364, 9.783) (1.4384, 9.8041) (1.4399, 9.8322) (1.44, 9.8676) (1.4389, 9.903) (1.437, 9.9385) (1.4347, 9.9741) (1.4321, 10.0097) (1.4292, 10.0453) (1.4258, 10.0808) (1.4228, 10.1092) (1.4202, 10.1304) (1.4184, 10.1446) (1.4175, 10.1515) knots 0 0 0 0 0 0 0.014286 0.028571 0.042857 0.057143 0.071429 0.085714 0.1 0.114286 0.128571 0.142857 0.156761 0.156761 0.156761 0.156761 0.156761 0.156761
  arc A33 (1.4175, 10.1515) -> (-1.4175, 10.1515) centre (0, 0) ccw
  spline S16 degree 5 poles (-1.4335, 9.7621) (-1.4345, 9.7691) (-1.4364, 9.783) (-1.4384, 9.8041) (-1.4399, 9.8322) (-1.44, 9.8676) (-1.4389, 9.903) (-1.437, 9.9385) (-1.4347, 9.9741) (-1.4321, 10.0097) (-1.4292, 10.0453) (-1.4258, 10.0808) (-1.4228, 10.1092) (-1.4202, 10.1304) (-1.4184, 10.1446) (-1.4175, 10.1515) knots 0 0 0 0 0 0 0.014286 0.028571 0.042857 0.057143 0.071429 0.085714 0.1 0.114286 0.128571 0.142857 0.156761 0.156761 0.156761 0.156761 0.156761 0.156761
  line L16 (-1.4335, 9.7621) -> (-1.3509, 9.1959)
  arc A34 (-2.0901, 8.0834) -> (-1.3509, 9.1959) centre (-2.3404, 9.0515) ccw
  arc A35 (-2.0901, 8.0834) -> (-2.2316, 8.0454) centre (0, 0) ccw
  arc A36 (-3.428, 8.6393) -> (-2.2316, 8.0454) centre (-2.4989, 9.0091) ccw
  line L17 (-3.428, 8.6393) -> (-3.6396, 9.171)
  spline S17 degree 5 poles (-3.6396, 9.171) (-3.6422, 9.1775) (-3.6476, 9.1905) (-3.6563, 9.2098) (-3.6691, 9.2349) (-3.6867, 9.2656) (-3.7054, 9.2957) (-3.7248, 9.3255) (-3.7446, 9.3552) (-3.7646, 9.3847) (-3.785, 9.4141) (-3.8056, 9.4432) (-3.8224, 9.4662) (-3.8353, 9.4833) (-3.8439, 9.4946) (-3.8482, 9.5002) knots 0 0 0 0 0 0 0.014286 0.028571 0.042857 0.057143 0.071429 0.085714 0.1 0.114286 0.128571 0.142857 0.156761 0.156761 0.156761 0.156761 0.156761 0.156761
  arc A37 (-3.8482, 9.5002) -> (-6.3033, 8.0827) centre (0, 0) ccw
  spline S18 degree 5 poles (-6.1225, 7.7374) (-6.1269, 7.743) (-6.1354, 7.7542) (-6.1477, 7.7714) (-6.1631, 7.795) (-6.1809, 7.8255) (-6.1976, 7.8568) (-6.2138, 7.8885) (-6.2295, 7.9205) (-6.2451, 7.9526) (-6.2604, 7.9849) (-6.2752, 8.0173) (-6.2868, 8.0434) (-6.2952, 8.0631) (-6.3006, 8.0763) (-6.3033, 8.0827) knots 0 0 0 0 0 0 0.014286 0.028571 0.042857 0.057143 0.071429 0.085714 0.1 0.114286 0.128571 0.142857 0.156761 0.156761 0.156761 0.156761 0.156761 0.156761
  line L18 (-6.1225, 7.7374) -> (-5.7679, 7.2884)
  arc A38 (-5.8518, 5.9553) -> (-5.7679, 7.2884) centre (-6.5526, 6.6686) ccw
  arc A39 (-5.8518, 5.9553) -> (-5.9553, 5.8518) centre (0, 0) ccw
  arc A40 (-7.2884, 5.7679) -> (-5.9553, 5.8518) centre (-6.6686, 6.5526) ccw
  line L19 (-7.2884, 5.7679) -> (-7.7374, 6.1225)
  spline S19 degree 5 poles (-7.7374, 6.1225) (-7.743, 6.1269) (-7.7542, 6.1354) (-7.7714, 6.1477) (-7.795, 6.1631) (-7.8255, 6.1809) (-7.8568, 6.1976) (-7.8885, 6.2138) (-7.9205, 6.2295) (-7.9526, 6.2451) (-7.9849, 6.2604) (-8.0173, 6.2752) (-8.0434, 6.2868) (-8.0631, 6.2952) (-8.0763, 6.3006) (-8.0827, 6.3033) knots 0 0 0 0 0 0 0.014286 0.028571 0.042857 0.057143 0.071429 0.085714 0.1 0.114286 0.128571 0.142857 0.156761 0.156761 0.156761 0.156761 0.156761 0.156761
  arc A41 (-8.0827, 6.3033) -> (-9.5002, 3.8482) centre (0, 0) ccw
  spline S20 degree 5 poles (-9.171, 3.6396) (-9.1775, 3.6422) (-9.1905, 3.6476) (-9.2098, 3.6563) (-9.2349, 3.6691) (-9.2656, 3.6867) (-9.2957, 3.7054) (-9.3255, 3.7248) (-9.3552, 3.7446) (-9.3847, 3.7646) (-9.4141, 3.785) (-9.4432, 3.8056) (-9.4662, 3.8224) (-9.4833, 3.8353) (-9.4946, 3.8439) (-9.5002, 3.8482) knots 0 0 0 0 0 0 0.014286 0.028571 0.042857 0.057143 0.071429 0.085714 0.1 0.114286 0.128571 0.142857 0.156761 0.156761 0.156761 0.156761 0.156761 0.156761
  line L20 (-9.171, 3.6396) -> (-8.6393, 3.428)
  arc A42 (-8.0454, 2.2316) -> (-8.6393, 3.428) centre (-9.0091, 2.4989) ccw
  arc A43 (-8.0454, 2.2316) -> (-8.0834, 2.0901) centre (0, 0) ccw
  arc A44 (-9.1959, 1.3509) -> (-8.0834, 2.0901) centre (-9.0515, 2.3404) ccw
  line L21 (-9.1959, 1.3509) -> (-9.7621, 1.4335)
  spline S21 degree 5 poles (-9.7621, 1.4335) (-9.7691, 1.4345) (-9.783, 1.4364) (-9.8041, 1.4384) (-9.8322, 1.4399) (-9.8676, 1.44) (-9.903, 1.4389) (-9.9385, 1.437) (-9.9741, 1.4347) (-10.0097, 1.4321) (-10.0453, 1.4292) (-10.0808, 1.4258) (-10.1092, 1.4228) (-10.1304, 1.4202) (-10.1446, 1.4184) (-10.1515, 1.4175) knots 0 0 0 0 0 0 0.014286 0.028571 0.042857 0.057143 0.071429 0.085714 0.1 0.114286 0.128571 0.142857 0.156761 0.156761 0.156761 0.156761 0.156761 0.156761
  arc A45 (-10.1515, 1.4175) -> (-10.1515, -1.4175) centre (0, 0) ccw
  spline S22 degree 5 poles (-9.7621, -1.4335) (-9.7691, -1.4345) (-9.783, -1.4364) (-9.8041, -1.4384) (-9.8322, -1.4399) (-9.8676, -1.44) (-9.903, -1.4389) (-9.9385, -1.437) (-9.9741, -1.4347) (-10.0097, -1.4321) (-10.0453, -1.4292) (-10.0808, -1.4258) (-10.1092, -1.4228) (-10.1304, -1.4202) (-10.1446, -1.4184) (-10.1515, -1.4175) knots 0 0 0 0 0 0 0.014286 0.028571 0.042857 0.057143 0.071429 0.085714 0.1 0.114286 0.128571 0.142857 0.156761 0.156761 0.156761 0.156761 0.156761 0.156761
  line L22 (-9.7621, -1.4335) -> (-9.1959, -1.3509)
  arc A46 (-8.0834, -2.0901) -> (-9.1959, -1.3509) centre (-9.0515, -2.3404) ccw
  arc A47 (-8.0834, -2.0901) -> (-8.0454, -2.2316) centre (0, 0) ccw
  arc A48 (-8.6393, -3.428) -> (-8.0454, -2.2316) centre (-9.0091, -2.4989) ccw
  line L23 (-8.6393, -3.428) -> (-9.171, -3.6396)
  spline S23 degree 5 poles (-9.171, -3.6396) (-9.1775, -3.6422) (-9.1905, -3.6476) (-9.2098, -3.6563) (-9.2349, -3.6691) (-9.2656, -3.6867) (-9.2957, -3.7054) (-9.3255, -3.7248) (-9.3552, -3.7446) (-9.3847, -3.7646) (-9.4141, -3.785) (-9.4432, -3.8056) (-9.4662, -3.8224) (-9.4833, -3.8353) (-9.4946, -3.8439) (-9.5002, -3.8482) knots 0 0 0 0 0 0 0.014286 0.028571 0.042857 0.057143 0.071429 0.085714 0.1 0.114286 0.128571 0.142857 0.156761 0.156761 0.156761 0.156761 0.156761 0.156761
  spline S24 degree 5 poles (-1.4335, 9.7621) (-1.4345, 9.7691) (-1.4364, 9.783) (-1.4384, 9.8041) (-1.4399, 9.8322) (-1.44, 9.8676) (-1.4389, 9.903) (-1.437, 9.9385) (-1.4347, 9.9741) (-1.4321, 10.0097) (-1.4292, 10.0453) (-1.4258, 10.081) (-1.422, 10.1167) (-1.4175, 10.1525) (-1.4124, 10.1882) (-1.4067, 10.224) (-1.4005, 10.2599) (-1.3939, 10.2957) (-1.387, 10.3316) (-1.3797, 10.3674) (-1.3721, 10.4033) (-1.364, 10.4391) (-1.3556, 10.475) (-1.3469, 10.5109) (-1.3377, 10.5468) (-1.3281, 10.5826) (-1.3182, 10.6185) (-1.3079, 10.6543) (-1.2973, 10.6902) (-1.2864, 10.726) (-1.2752, 10.7619) (-1.2636, 10.7977) (-1.2517, 10.8335) (-1.2395, 10.8693) (-1.227, 10.905) (-1.2141, 10.9408) (-1.2009, 10.9765) (-1.1875, 11.0122) (-1.1737, 11.0479) (-1.1597, 11.0835) (-1.1453, 11.1191) (-1.1307, 11.1547) (-1.1158, 11.1903) (-1.1005, 11.2259) (-1.085, 11.2614) (-1.0692, 11.2968) (-1.0532, 11.3323) (-1.0368, 11.3677) (-1.0202, 11.4031) (-1.0033, 11.4384) (-0.9861, 11.4737) (-0.9687, 11.5089) (-0.951, 11.5441) (-0.933, 11.5793) (-0.9148, 11.6144) (-0.8963, 11.6495) (-0.8775, 11.6845) (-0.8585, 11.7195) (-0.8392, 11.7545) (-0.8197, 11.7894) (-0.7999, 11.8242) (-0.7799, 11.859) (-0.7596, 11.8937) (-0.7391, 11.9284) (-0.7183, 11.963) (-0.6972, 11.9976) (-0.6759, 12.0321) (-0.6544, 12.0666) (-0.6327, 12.101) (-0.6106, 12.1353) (-0.5884, 12.1696) (-0.5704, 12.197) (-0.5568, 12.2175) (-0.5477, 12.2311) (-0.5431, 12.238) knots 0 0 0 0 0 0 0.01428571 0.02857143 0.04285714 0.05714286 0.07142857 0.08571429 0.1 0.11428571 0.12857143 0.14285714 0.15714286 0.17142857 0.18571429 0.2 0.21428571 0.22857143 0.24285714 0.25714286 0.27142857 0.28571429 0.3 0.31428571 0.32857143 0.34285714 0.35714286 0.37142857 0.38571429 0.4 0.41428571 0.42857143 0.44285714 0.45714286 0.47142857 0.48571429 0.5 0.51428571 0.52857143 0.54285714 0.55714286 0.57142857 0.58571429 0.6 0.61428571 0.62857143 0.64285714 0.65714286 0.67142857 0.68571429 0.7 0.71428571 0.72857143 0.74285714 0.75714286 0.77142857 0.78571429 0.8 0.81428571 0.82857143 0.84285714 0.85714286 0.87142857 0.88571429 0.9 0.91428571 0.92857143 0.94285714 0.95714286 0.97142857 0.98571429 1 1 1 1 1 1
  circle A49 centre (0, 0) radius 10.5
  line L24 (0, 0) -> (-1.3705, 10.4102)
  line L25 (0, 0) -> (0, 13) construction
  spline S25 degree 3 poles (-5.6486, 10.8699) (-4.6241, 10.3659) (-4.0866, 9.8097) (-3.8482, 9.5002) knots -0.162759 -0.162759 -0.162759 -0.162759 0 0 0 0
  line L26 (-4.0175, 9.701) -> (0, 0)
  point P0 (-1.3705, 10.4102)
  point P1 (-4.0175, 9.701)
  constraint coincident P0 S24
  constraint coincident P0 A49
  constraint coincident A0.centre A1.centre
  constraint coincident P0 L24.end
  constraint vertical L25
  constraint coincident P1 S25
  constraint coincident A49 P1
  constraint coincident P1 L26.start
extrude "Extrude5" add 1 faces at (0.2558, 0.8292, 0) along direction (0, 0, 1) blind 6 in component "Spur Gear (12 teeth)"